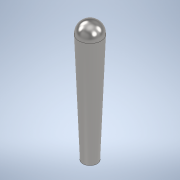
# Autodesk Inventor part: switch_stem
Saved by Autodesk Inventor 2022.2 (Build 262287000, 287)
## iProperties
Created: 2022-01-24
Part Number: switch_stem
Material: Stainless Steel
Document SubType Name: Modeling
Designer: hugof
Density: 8 g/cm^3
Appearance: Semi-Polished
Author: hugof
Autodesk Inventor part; units mm, degrees
ref_plane "YZ Plane" through (0, 0, 0) normal (1, 0, 0) x (0, 1, 0)
ref_plane "XZ Plane" through (0, 0, 0) normal (0, 1, 0) x (-1, 0, 0)
ref_plane "XY Plane" through (0, 0, 0) normal (0, 0, 1) x (1, 0, 0)
sketch "Sketch1" plane through (0, 0, 0) normal (0, 0, 1) x (1, 0, 0)
  line L0 (0, 0) -> (0.95, 0)
  line L1 (0.95, 0) -> (1.5, 14.5)
  line L2 (0, 0) -> (0, 14.5)
  line L3 (0, 14.5) -> (1.5, 14.5)
  dimension "d0" = 14.5
  dimension "d1" = 0.95
  dimension "d2" = 1.5
  constraints: 8 end point, 1 horizontal, 1 perpendicular, 1 vertical
  measures "d0" distance of L0.start L2.end
  measures "d1" distance of L0.start L0.end
  measures "d2" distance of L2.end L1.end
revolve "Revolution1" add sketch "Sketch1" angle 360 about axis through (0, 0, 0) along (0, 1, 0)
sketch "Sketch2" plane through (0, 14.5, 0) normal (0, 1, 0) x (1, 0, 0)
  circle A0 centre (0, 0) radius 1.5
  circle A1 centre (0, 0) radius 1.5 projected
  line L0 (-0.9881, -1.1286) -> (0.9881, 1.1286)
  constraints: 2 end point, 2 point on circle, 1 centre point, 1 coincident, 1 midpoint, 2 other
revolve "Revolution2" add sketch "Sketch2" angle 360 about axis through (-0.9881, 14.5, 1.1286) along (0.6587096, 0, -0.7523973) picked at (0.7723, -0.1849) contours A0 L0
body "Solid1"
